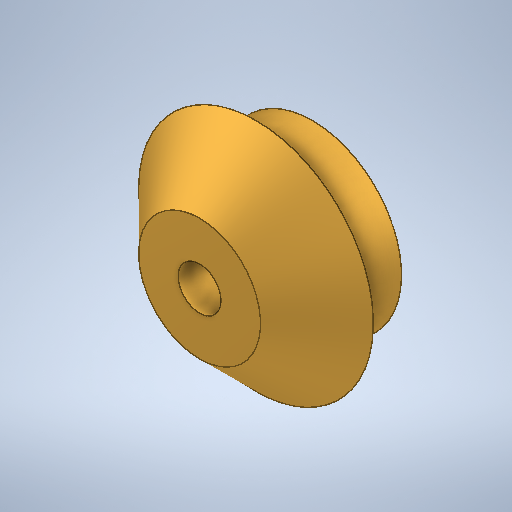
# Autodesk Inventor part: guide
Saved by Autodesk Inventor 2025.1 (Build 291241000, 241)
## iProperties
Created: 2025-03-11
Part Number: guide
Material: Generic
Document SubType Name: Modeling
Designer: santiago
Density: 1 g/cm^3
Appearance: Brass - Satin
Author: santiago
Autodesk Inventor part; units mm, degrees
ref_plane "YZ Plane" through (0, 0, 0) normal (1, 0, 0) x (0, 1, 0)
ref_plane "XY Plane" through (0, 0, 0) normal (0, 0, 1) x (1, 0, 0)
sketch "Sketch1" plane through (0, 0, 0) normal (1, 0, 0) x (0, 1, 0)
  line L0 (0.0289, 5.9359) -> (3.5289, 5.9359)
  line L1 (-1.8711, 5.9359) -> (-1.8711, -4.0641) construction
  line L2 (6.0289, 0.9359) -> (8.5289, 0.9359)
  line L3 (3.5289, 5.9359) -> (8.5289, 0.9359)
  line L4 (0.0289, -4.0641) -> (6.0289, -4.0641)
  line L5 (6.0289, -4.0641) -> (6.0289, 0.9359)
  line L6 (0.0289, 5.9359) -> (0.0289, -0.0641)
  line L7 (0.0289, -0.0641) -> (-1.8711, -0.0641)
  line L8 (-1.8711, -4.0641) -> (0.0289, -4.0641)
  line L9 (-1.8711, -0.0641) -> (-1.8711, -4.0641)
  point P0 (0, 0)
  dimension "d0" = 3.5
  dimension "d3" = 10
  dimension "d11" = 6
  constraints: 20 end point, 3 horizontal, 2 perpendicular, 2 vertical, 1 collinear, 1 parallel, 1 point on line
  measures "d0" distance of L0.start L0.end
  measures "d3" distance of L0.start L4.start
  measures "d11" distance of L0.start L6.end
revolve "Revolution1" add sketch "Sketch1" angle 360 about axis through (0, -1.8711, 5.9359) along (0, 0, -1)
ref_plane "Work Plane1" through (0, 6.0289, -1.5641) normal (0, 1, 0) x (-1, 0, 0)
body "Solid1"
